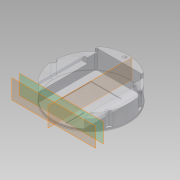
# Autodesk Inventor part: bottom1_2_bigtouch
Saved by Autodesk Inventor 2015 SP2 (Build 190223200, 223)
## iProperties
Created: 2015-01-05
Part Number: bottom1_2_bigtouch
Material: Acrylic
Document SubType Name: Modeling
Designer: Mathieu
Density: 1.188 g/cm^3
Appearance: Transparent - Clear
Mass: 1.2332 g
Surface Area: 16.4283 cm^2
Volume: 1.03804 cm^3
Author: Mathieu
Autodesk Inventor part; units mm, degrees
ref_plane "YZ Plane" through (0, 0, 0) normal (1, 0, 0) x (0, 1, 0)
ref_plane "XZ Plane" through (0, 0, 0) normal (0, 1, 0) x (-1, 0, 0)
ref_plane "XY Plane" through (0, 0, 0) normal (0, 0, 1) x (1, 0, 0)
sketch "Sketch1" plane through (0, 0, 0) normal (0, 0, 1) x (1, 0, 0)
  line L0 (-3.8177, -2.5414) -> (-3.8177, 2.9086)
  line L1 (-3.8177, 2.9086) -> (8.4464, 2.9086)
  line L2 (8.4323, 2.6586) -> (8.4323, -2.5414)
  line L3 (8.4323, -2.5414) -> (-3.8177, -2.5414)
  line L4 (-3.8177, 8.4062) -> (-3.8177, -10.1402)
  line L5 (8.4323, 2.6586) -> (8.5573, 2.9086)
  line L6 (8.5573, 2.9086) -> (8.4464, 2.9086)
  point P0 (0, 0)
  dimension "d1" = 24.5
  dimension "d2" = 5.45
  dimension "d29" = 0.25
  dimension "d30" = 24.75
  constraints: 14 end point, 3 perpendicular, 2 collinear, 2 vertical
  measures "d1" diameter of L2 L4
  measures "d2" distance of L1.end L2.end
  measures "d29" distance from line of L2.start L1
  measures "d30" diameter of L5.end L4
revolve "Revolution1" add sketch "Sketch1" angle 360 about axis through (-3.8177, 8.4062, 0) along (0, -1, 0)
sketch "Sketch2" plane through (-3.8177, -2.5414, 0) normal (0, -1, 0) x (1, 0, 0)
  circle A0 centre (0, 0) radius 12.75 construction
  circle A1 centre (0, 0) radius 12.25 projected
  line L0 (0, 12.75) -> (0, -12.75) construction
  line L1 (-5.3884, -11.5554) -> (5.3884, 11.5554) construction
  line L2 (-5.3884, 11.5554) -> (5.3884, -11.5554) construction
  circle A2 centre (-5.3884, -11.5554) radius 1.1
  circle A3 centre (5.3884, -11.5554) radius 1.1
  circle A4 centre (0, 12.75) radius 1.1
  point P0 (3.8177, 0)
  dimension "d4" = 25.5
  dimension "d5" = 25
  dimension "d6" = 25
  dimension "d7" = 2.2
  constraints: 6 end point, 6 point on circle, 5 midpoint, 4 centre point, 3 coincident, 2 equal radius, 1 concentric, 1 vertical
  measures "d4" diameter of A0
  measures "d5" angle of L2 L0
  measures "d6" angle of L0 L1
  measures "d7" diameter of A4
extrude "Extrusion1" cut sketch "Sketch2" against normal blind 4.75 contours A4 A1 | A1 A4 | A3 A1 | A1 A3 | A2 A1 | A1 A2
sketch "Sketch3" plane through (-3.8177, -2.5414, 0) normal (0, -1, 0) x (1, 0, 0)
  line L0 (-12.375, -7.5) -> (9.1567, -7.5)
  line L1 (9.1567, 7.5) -> (-12.375, 7.5)
  circle A0 centre (0, 0) radius 9.9629 construction
  line L2 (-12.375, 7.5) -> (-12.375, -7.5)
  line L3 (9.1567, -7.5) -> (9.1567, 7.5)
  circle A1 centre (0, 0) radius 12.375 projected
  point P0 (-9.8433, -7.5)
  dimension "d11" = 15
  dimension "d92" = 7.5
  dimension "d94" = 19
  constraints: 8 end point, 2 parallel, 1 centre point, 1 horizontal, 1 perpendicular, 1 point on line, 1 vertical, 3 other
  measures "d11" distance of L1.start L0.end
  measures "d92" distance from line of A0.centre L0
  measures "d94" distance from line of L3 point (-9.843, -7.5)
extrude "Extrusion2" cut sketch "Sketch3" against normal up to surface (4.75 mm away) contours L2 A1 L0 | A1 L1 L3 L0 | L2 L1 A1 picked at (1.9795, 0)
sketch "Sketch5" plane through (-13.5034, 2.2086, 7.5) normal (0, -1, 0) x (1, 0, 0)
  line L0 (14.6857, -2.5) -> (4.6857, -2.5)
  line L1 (4.6857, -2.5) -> (4.6857, -12.5)
  line L2 (4.6857, -12.5) -> (14.6857, -12.5)
  line L3 (14.6857, -12.5) -> (14.6857, -2.5)
  line L4 (14.6857, -2.5) -> (4.6857, -12.5) construction
  line L5 (4.6857, -2.5) -> (14.6857, -12.5) construction
  line L6 (-1.8929, -11.5) -> (-2.0018, -11.5)
  arc A0 (0, 0) -> (0, -15) centre (9.6857, -7.5) ccw projected
  arc A1 (0.7907, -0.6122) -> (0.7907, -14.3878) centre (9.6857, -7.5) ccw
  line L7 (4.6857, -11.25) -> (-0.9209, -11.25)
  line L8 (-1.223, -10.25) -> (4.6857, -10.25)
  point P0 (4.6857, -11.5)
  dimension "d95" = 10
  dimension "d99" = 1
  dimension "d100" = 1
  dimension "d101" = 1.25
  constraints: 18 end point, 4 point on circle, 3 horizontal, 3 midpoint, 3 perpendicular, 3 point on line, 2 parallel, 1 centre point, 1 coincident
  measures "d95" distance of L0.start L0.end
  measures "d99" radial gap between concentric circles of A1 A0
  measures "d100" distance between parallel lines of L8 L7
  measures "d101" distance between parallel lines of L2 L7
extrude "Extrusion3" cut sketch "Sketch5" against normal blind 0.25
sketch "Sketch7" plane through (-3.8177, 2.9086, 0) normal (0, 1, 0) x (1, 0, 0)
  arc A0 (12.3346, 0.9992) -> (12.3346, -0.9992) centre (12.375, 0) ccw
  circle A1 centre (0, 0) radius 12.375 projected
  arc A2 (-12.3346, -0.9992) -> (-12.3346, 0.9992) centre (-12.375, 0) ccw
  line L0 (-12.375, 0) -> (12.375, 0) construction
  dimension "d34" = 2
  constraints: 10 point on circle, 2 centre point, 2 end point, 1 coincident, 1 equal radius, 1 horizontal, 1 midpoint
  measures "d34" diameter of A2
extrude "Extrusion5" [suppressed]
ref_plane "Work Plane1" through (-13.5034, 0.0586, -7.5) normal (1, 0, 0) x (0, 1, 0)
ref_plane "Work Plane3" through (-16.0677, 0.0586, 0) normal (-1, 0, 0) x (0, -1, 0)
ref_plane "Work Plane2" through (5.339, -2.5414, 0) normal (0, 0, -1) x (-1, 0, 0)
sketch "Sketch10" plane through (-13.5034, 0.0586, -7.5) normal (1, 0, 0) x (0, 1, 0)
  line L0 (-0.8679, 15) -> (-0.8679, 17)
  line L1 (-0.8679, 17) -> (-2.6, 16)
  line L2 (2.15, 15) -> (-2.6, 15) projected
  line L3 (-2.6, 19.7124) -> (-2.6, 15) projected
  line L4 (-2.6, 0) -> (2.15, 0) projected
  line L5 (-2.6, 0) -> (-2.6, -3.1626) projected
  point P0 (-0.0586, 7.5)
  dimension "d69" = 60
  dimension "d70" = 1
  dimension "d71" = 2
  constraints: 4 end point, 2 point on line, 1 vertical
  measures "d69" angle of L0 L1
  measures "d70" distance from line of L2 L1.end
  measures "d71" distance of L0.start L0.end
extrude "Extrusion8" cut sketch "Sketch10" along normal blind 16
mirror "Mirror1" about plane through (5.339, -2.5414, 0) normal (0, 0, -1) of "Extrusion8"
chamfer "Chamfer2" distance 0.25 angle 45 3 edges at (-8.7412, -2.5414, -10.5585) (1.1058, -2.5414, -10.5585) (-3.8177, -2.5414, 11.65)
sketch "Sketch11" plane through (5.339, -2.5414, -7.5) normal (0, -1, 0) x (1, 0, 0)
  arc A0 (-10.3843, 19.6883) -> (-7.9291, 19.6883) centre (-9.1567, 20.25) ccw projected
  arc A1 (-10.3843, 19.6883) -> (-17.9778, 16) centre (-9.1567, 7.5) ccw projected
  line L0 (-17.9778, 16) -> (-2.8424, 16) projected
  line L1 (-2.8424, 16) -> (-2.8424, 15) projected
  line L2 (-2.8424, 15) -> (0, 15) projected
  line L3 (0, 15) -> (0, 0) projected
  line L4 (0, 0) -> (-2.8424, 0) projected
  line L5 (-2.8424, 0) -> (-2.8424, -1) projected
  line L6 (-2.8424, -1) -> (-17.9778, -1) projected
  arc A2 (-17.9778, -1) -> (-15.4203, -3.0276) centre (-9.1567, 7.5) ccw projected
  arc A3 (-13.1951, -4.0652) -> (-15.4203, -3.0276) centre (-14.5451, -4.0554) ccw projected
  arc A4 (-13.1951, -4.0652) -> (-5.1183, -4.0652) centre (-9.1567, 7.5) ccw projected
  arc A5 (-2.8931, -3.0276) -> (-5.1183, -4.0652) centre (-3.7683, -4.0554) ccw projected
  arc A6 (-2.8931, -3.0276) -> (-7.9291, 19.6883) centre (-9.1567, 7.5) ccw projected
  line L7 (0, 0.1) -> (0.6056, 0.1)
  line L8 (0, 14.9) -> (0.6056, 14.9)
  line L9 (-18.8424, 0) -> (-2.8424, 0) projected
  dimension "d82" = 0.1
  dimension "d83" = 0.1
  constraints: 4 end point, 2 horizontal, 2 point on circle, 2 point on line
  measures "d82" distance between parallel lines of L2 L8
  measures "d83" distance between parallel lines of L9 L7
extrude "Extrusion9" add sketch "Sketch11" along normal blind 1.5 contours A6 L7 L3 L8
chamfer "Chamfer3" distance 0.5 angle 45 2 edges at (5.339, -0.1664, 7.5) (5.339, -0.1664, -7.5)
sketch "Sketch12" plane through (5.339, -4.0414, -7.5) normal (0, -1, 0) x (1, 0, 0)
  circle A0 centre (1.8433, 7.5) radius 0.4
  circle A1 centre (-9.1567, 7.5) radius 12.25 construction
  arc A2 (-13.1951, -4.0652) -> (-5.1183, -4.0652) centre (-9.1567, 7.5) ccw projected
  dimension "d87" = 11
  dimension "d88" = 0.8
  constraints: 2 centre point, 2 concentric, 1 horizontal alignment
  measures "d87" distance of A0.centre A1.centre
  measures "d88" diameter of A0
extrude "Extrusion10" add sketch "Sketch12" along normal blind 0.3
fillet "Fillet1" radius 0.25 2 edges at (6.7823, -4.0414, 0) (6.7823, -4.3414, 0)
equation "\"d92\" = 0.5 * d11"
body "Solid1"
